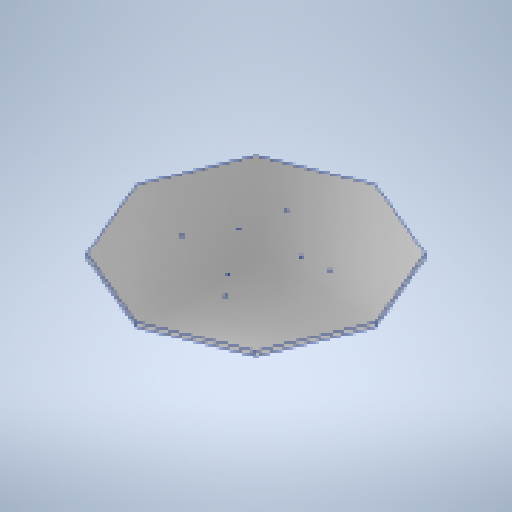
# Autodesk Inventor part: Largebaseplate
Saved by Autodesk Inventor 2024.3 (Build 283343010, 343A)
## iProperties
Created: 2025-05-29
Part Number: Largebaseplate
Material: アルミニウム 6061
Document SubType Name: Modeling
Designer: kshau
Density: 2.7 g/cm^3
Appearance: アルミニウム - フラット
Author: kshau
Autodesk Inventor part; units mm, degrees
ref_plane "YZ Plane" through (0, 0, 0) normal (1, 0, 0) x (0, 1, 0)
ref_plane "XZ Plane" through (0, 0, 0) normal (0, 1, 0) x (-1, 0, 0)
ref_plane "XY Plane" through (0, 0, 0) normal (0, 0, 1) x (1, 0, 0)
sketch "スケッチ1" plane through (0, 0, 0) normal (0, 1, 0) x (-1, 0, 0)
  circle A0 centre (0, 0) radius 135.299
  line L0 (0, 0) -> (135.299, 0)
  line L1 (0, 0) -> (95.6709, -95.6709)
  line L2 (0, 0) -> (0, -135.299)
  line L3 (0, 0) -> (-95.6709, -95.6709)
  line L4 (0, 0) -> (-135.299, 0)
  line L5 (0, 0) -> (-95.6709, 95.6709)
  line L6 (0, 0) -> (0, 135.299)
  line L7 (0, 0) -> (95.6709, 95.6709)
  line L8 (135.299, 0) -> (95.6709, -95.6709)
  line L9 (95.6709, 95.6709) -> (135.299, 0)
  line L10 (0, 135.299) -> (95.6709, 95.6709)
  line L11 (-95.6709, 95.6709) -> (0, 135.299)
  line L12 (-135.299, 0) -> (-95.6709, 95.6709)
  line L13 (-95.6709, -95.6709) -> (-135.299, 0)
  line L14 (0, -135.299) -> (-95.6709, -95.6709)
  line L15 (95.6709, -95.6709) -> (0, -135.299)
  circle A1 centre (0, 0) radius 125
  point P0 (0, 135.299)
  point P1 (-95.6709, 95.6709)
  point P2 (-135.299, 0)
  point P3 (95.6709, -95.6709)
  dimension "d3" = 360
  dimension "d7" = 360
  dimension "d57" = 250
  constraints: 32 end point, 2 coincident, 1 centre point, 1 horizontal, 1 horizontal alignment, 1 tangent, 52 other
  measures "d57" diameter of A1
extrude "押し出し1" add sketch "スケッチ1" along normal blind 5 contours L8 A1 L0 | L0 A1 L9 | L9 A1 L7 | L7 A1 L10 | L15 A1 L1 | L1 A1 L8 | A1 L1 L0 | L0 L7 A1 | L10 A1 L6 | L6 A1 L11 | L7 L6 A1 | L14 A1 L2 | L2 A1 L15 | A1 L2 L1 | L2 A1 L3 | L3 A1 L4 | L4 A1 L5 | L5 A1 L6 | L11 A1 L5 | L5 A1 L12 | L13 A1 L3 | L3 A1 L14 | A1 L13 L4 | L4 L12 A1
sketch "スケッチ2" plane through (0, 5, 0) normal (0, 1, 0) x (1, 0, 0)
  circle A0 centre (0, 0) radius 64
  circle A1 centre (0, 0) radius 36.5
  line L0 (0, 0) -> (-59.1283, 24.4917)
  line L1 (-95.6709, 95.6709) -> (-135.299, 0) projected
  line L2 (0, 0) -> (-135.299, 0)
  point P0 (-33.7216, 13.9679)
  point P1 (4.7642, -36.1877)
  point P2 (28.9574, 22.2198)
  dimension "d11" = 128
  dimension "d12" = 73
  dimension "d13" = 22.5
  dimension "d16" = 360
  constraints: 4 end point, 2 coincident, 1 horizontal, 1 point on line, 10 other
  measures "d13" angle of L2 L0
hole "穴1" at (-33.7216, 5, -13.9679) at (4.7642, 5, 36.1877) at (28.9574, 5, -22.2198) direction (0, -1, 0) diameter 3.2 end through all
sketch "スケッチ3" plane through (0, 5, 0) normal (0, 1, 0) x (1, 0, 0)
  circle A0 centre (0, 0) radius 64
  line L0 (0, 0) -> (-59.1283, -24.4917)
  line L1 (0, 0) -> (-29.4133, 0)
  point P0 (-59.1283, -24.4917)
  point P1 (24.4917, -59.1283)
  point P2 (59.1283, 24.4917)
  point P3 (-24.4917, 59.1283)
  dimension "d25" = 128
  dimension "d28" = 360
  dimension "d56" = 22.5
  constraints: 4 end point, 2 point on circle, 1 centre point, 1 coincident, 1 horizontal, 1 point on line, 5 other
  measures "d25" diameter of A0
  measures "d56" angle of L1 L0
hole "穴2" at (-59.1283, 5, 24.4917) at (24.4917, 5, 59.1283) at (59.1283, 5, -24.4917) at (-24.4917, 5, -59.1283) direction (0, -1, 0) diameter 3.2 end through all
sketch "スケッチ4" plane through (0, 0, 0) normal (0, -1, 0) x (1, 0, 0)
  circle A0 centre (-33.7216, -13.9679) radius 1.6 projected
  circle A1 centre (-33.7216, -13.9679) radius 3
  circle A2 centre (28.9574, -22.2198) radius 3
  circle A3 centre (4.7642, 36.1877) radius 3
  circle A4 centre (-24.4917, -59.1283) radius 1.6 projected
  circle A5 centre (-24.4917, -59.1283) radius 3.9
  circle A6 centre (59.1283, -24.4917) radius 3.9
  circle A7 centre (24.4917, 59.1283) radius 3.9
  circle A8 centre (-59.1283, 24.4917) radius 3.9
  point P0 (0, 0)
  point P1 (0, 0)
  point P2 (0, 0)
  dimension "d37" = 6
  dimension "d40" = 360
  dimension "d42" = 7.8
  dimension "d45" = 360
  constraints: 7 centre point, 4 coincident, 17 other
  measures "d37" diameter of A1
  measures "d42" diameter of A5
extrude "押し出し2" [suppressed]
sketch "スケッチ5" plane through (0, 0, 0) normal (0, -1, 0) x (1, 0, 0)
  circle A0 centre (59.1283, -24.4917) radius 1.6 projected
  circle A1 centre (59.1283, -24.4917) radius 3.9
  circle A2 centre (24.4917, 59.1283) radius 3.9
  circle A3 centre (-59.1283, 24.4917) radius 3.9
  circle A4 centre (-24.4917, -59.1283) radius 3.9
  point P0 (0, 0)
  dimension "d49" = 7.8
  dimension "d52" = 360
  constraints: 4 centre point, 1 coincident, 9 other
  measures "d49" diameter of A1
extrude "押し出し3" [suppressed]
sketch "スケッチ6" plane through (0, 0, 0) normal (0, -1, 0) x (1, 0, 0)
  line L0 (0, 0) -> (115.4849, 47.8354)
  line L1 (95.6709, 95.6709) -> (135.299, 0) projected
  line L2 (0, 135.299) -> (95.6709, 95.6709) projected
  line L3 (58.7953, 110.9452) -> (-120.0247, 36.8755)
  line L4 (-135.299, 0) -> (-95.6709, 95.6709) projected
  line L5 (-95.6709, 95.6709) -> (0, 135.299) projected
  line L6 (135.299, 0) -> (95.6709, -95.6709) projected
  line L7 (120.0247, -36.8755) -> (-58.7953, -110.9452)
  line L8 (0, -135.299) -> (-95.6709, -95.6709) projected
  line L9 (95.6709, -95.6709) -> (0, -135.299) projected
  line L10 (0, 0) -> (-30.6147, 73.9104)
  point P0 (43.2957, 104.525)
  point P1 (-104.525, 43.2957)
  point P2 (104.525, -43.2957)
  point P3 (-43.2957, -104.525)
  dimension "d58" = 80
  dimension "d59" = 80
  dimension "d60" = 80
  constraints: 8 end point, 5 point on line, 3 parallel, 3 symmetric about line, 2 midpoint
  measures "d58" distance between parallel lines of L0 L3
  measures "d59" distance between parallel lines of L0 L7
  measures "d60" distance from line of L10 point (43.296, 104.525)
hole "穴3" at (43.2957, 0, 104.525) at (-104.525, 0, 43.2957) at (104.525, 0, -43.2957) at (-43.2957, 0, -104.525) direction (0, 1, 0) diameter 3.1 end through all
